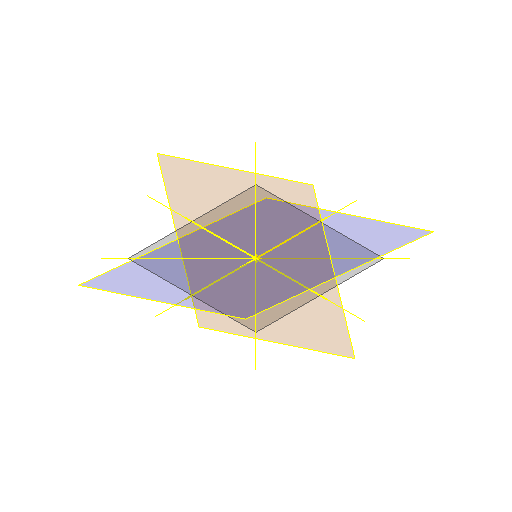
# Autodesk Inventor part: deflection_plane
Saved by Autodesk Inventor 2026.1 (Build 301233000, 233)
## iProperties
Created: 2025-08-08
Part Number: deflection_plane
Material: Generic
Document SubType Name: Modeling
Designer: farin012
Density: 1 g/cm^3
Appearance: Default
Author: farin012
Autodesk Inventor part; units mm, degrees
ref_plane "YZ Plane" through (0, 0, 0) normal (1, 0, 0) x (0, 1, 0)
sketch "Sketch1" plane through (0, 0, 0) normal (0, 1, 0) x (-1, 0, 0)
  line L0 (-8, 8) -> (8, 8)
  line L1 (8, 8) -> (8, -8)
  line L2 (8, -8) -> (-8, -8)
  line L3 (-8, -8) -> (-8, 8)
  line L4 (-8, 8) -> (8, -8) construction
  line L5 (8, 8) -> (-8, -8) construction
  point P0 (0, 0)
  dimension "d0" = 16
  dimension "d1" = 16
  constraints: 12 end point, 2 midpoint, 2 parallel, 1 horizontal, 1 perpendicular
  measures "d0" distance of L1.end L2.end
  measures "d1" distance of L0.end L1.end
extrude "Extrusion1" add sketch "Sketch1" along normal blind 0.0005
sketch "Sketch2" plane through (0, 0, 0) normal (0, -1, 0) x (1, 0, 0)
  line L0 (8, -8) -> (-8, -8) projected
  line L1 (-8, 8) -> (8, 8)
  line L2 (8, 8) -> (8, -8)
  line L3 (8, -8) -> (-8, -8)
  line L4 (-8, -8) -> (-8, 8)
  line L5 (-8, 8) -> (8, -8) construction
  line L6 (8, 8) -> (-8, -8) construction
  point P0 (0, 0)
  constraints: 12 end point, 2 midpoint, 2 parallel, 1 horizontal, 1 perpendicular
extrude "Extrusion2" add sketch "Sketch2" along normal blind 0.0005
ref_plane "Work Plane2" through (0, 0, 0) normal (0, 1, 0) x (1, 0, 0)
ref_plane "Work Plane3" through (0, 0, 0) normal (0, 0, 1) x (1, 0, 0)
ref_plane "Work Plane1" through (0, 0, 0) normal (-1, 0, 0) x (0, 0, -1)
sketch "Sketch4" plane through (0, 0, 0) normal (0, 0, 1) x (1, 0, 0)
  line L0 (0, 0) -> (-1.8844, 5.7996)
  line L1 (0, 0) -> (6.098, 0) construction
  line L2 (0, 0) -> (1.7067, -5.2527)
  line L3 (0, 0) -> (5.523, 0) construction
  dimension "d12" = 108
  dimension "d13" = 72
  constraints: 8 end point, 2 equal length, 2 horizontal
  measures "d12" angle of L1 L0
  measures "d13" angle of L2 L3
ref_plane "Work Plane8" through (0, 0, 0) normal (-0.309, 0.9511, 0) x (-0.9511, -0.309, 0)
ref_plane "Work Plane10" through (0, 0, 0) normal (0.9511, 0.309, 0) x (-0.309, 0.9511, 0)
ref_plane "Work Plane9" through (0, 0, 0) normal (0, 0, 1) x (-0.309, 0.9511, 0)
sketch "Sketch5" plane through (0, 0, 0) normal (0.9511, 0.309, 0) x (-0.309, 0.9511, 0)
  line L0 (0, 0) -> (-5.1358, 0.4042)
  line L1 (0, 0) -> (5.1517, 0) construction
  dimension "d15" = 175.5
  constraints: 4 end point, 1 equal length, 1 horizontal
  measures "d15" angle of L1 L0
ref_plane "Work Plane11" through (0, 0, 0) normal (0.3081, -0.9481, 0.0785) x (0.9511, 0.309, 0)
body "Solid1"
